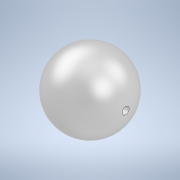
# Autodesk Inventor part: Ball
Saved by Autodesk Inventor 2021.1 (Build 251245010, 245A)
## iProperties
Created: 2025-09-17
Material: Stainless Steel
Document SubType Name: Modeling
Designer: SD
Density: 8 g/cm^3
Appearance: Semi-Polished
Mass: 2.14466 g
Surface Area: 2.01062 cm^2
Volume: 0.268083 cm^3
Project: Automatic Tea Steeping mechanism
Part Number: Ball
BOM-Mass: 0.00214
BOM-Area: 0.000
Diameter: 10.000 mm
Author: SD
Title: Ball
Autodesk Inventor part; units mm, degrees
ref_plane "YZ Plane" through (0, 0, 0) normal (1, 0, 0) x (0, 1, 0)
ref_plane "XZ Plane" through (0, 0, 0) normal (0, 1, 0) x (-1, 0, 0)
ref_plane "XY Plane" through (0, 0, 0) normal (0, 0, 1) x (1, 0, 0)
sketch "Sketch3" plane through (0, 0, 0) normal (0, 0, 1) x (1, 0, 0)
  line L0 (0, 0) -> (0, -10)
  arc A0 (0, -10) -> (0, 0) centre (0, -5) ccw
  line L1 (0, -5) -> (-0.832, -5) construction
  dimension "d23" = 10
  constraints: 4 end point, 2 point on circle, 1 centre point, 1 coincident, 1 horizontal, 1 midpoint, 1 vertical
  measures "d23" distance of L0.start L0.end
revolve "Revolution2" add sketch "Sketch3" angle 360 about axis through (0, 0, 0) along (0, -1, 0)
sketch "Sketch4" plane through (0, 0, 0) normal (1, 0, 0) x (0, 1, 0)
  circle A0 centre (-5, 0) radius 0.5
  point P0 (0, 0)
  dimension "d26" = 1
  dimension "d27" = 5
  constraints: 1 centre point, 1 horizontal alignment
  measures "d26" diameter of A0
  measures "d27" distance of A0.centre point (0, 0)
extrude "Extrusion1" cut sketch "Sketch4" along normal mid plane 10
body "Solid2"
